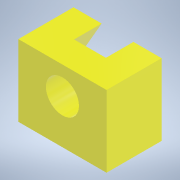
# Autodesk Inventor part: 2x 2x M6 Nut Holder
Saved by Autodesk Inventor 2022 (Build 260153000, 153)
## iProperties
Created: 2021-06-21
Part Number: 2x 2x M6 Nut Holder
Material: ABS Plastic
Document SubType Name: Modeling
Designer: benka
Density: 1.06 g/cm^3
Appearance: Yellow
Author: benka
Autodesk Inventor part; units mm, degrees
ref_plane "YZ Plane" through (0, 0, 0) normal (1, 0, 0) x (0, 1, 0)
ref_plane "XZ Plane" through (0, 0, 0) normal (0, 1, 0) x (-1, 0, 0)
ref_plane "XY Plane" through (0, 0, 0) normal (0, 0, 1) x (1, 0, 0)
sketch "Sketch1" plane through (0, 1.5, 0) normal (0, 0, 1) x (1, 0, 0)
  line L0 (8, 5) -> (8, -8)
  line L1 (8, -8) -> (-8, -8)
  line L2 (-8, -8) -> (-8, 5)
  line L3 (-8, 5) -> (8, 5)
  line L4 (-4.3301, 2.5) -> (-5.7735, 0)
  line L5 (-5.7735, 0) -> (-4.3301, -2.5)
  line L6 (-4.3301, -2.5) -> (-2.8868, -5)
  line L7 (-2.8868, -5) -> (0, -5)
  line L8 (0, -5) -> (2.8868, -5)
  line L9 (2.8868, -5) -> (4.3301, -2.5)
  line L10 (4.3301, -2.5) -> (5.7735, 0)
  line L11 (5.7735, 0) -> (4.3301, 2.5)
  line L12 (4.3301, 2.5) -> (2.8868, 5)
  line L13 (-2.8868, 5) -> (-4.3301, 2.5)
  point P0 (0, 0)
  constraints: 28 end point, 1 parallel, 1 perpendicular
extrude "Extrusion1" add sketch "Sketch1" along normal blind 5 contours L0 L1 L2 L3 L13 L4 L5 L6 L7 L8 L9 L10 L11 L12
sketch "Sketch2" plane through (0, 1.5, 5) normal (0, 0, 1) x (1, 0, 0)
  line L0 (-8, 5) -> (-8, -8) projected
  line L1 (8, 5) -> (-8, 5) projected
  line L2 (8, -8) -> (8, 5) projected
  line L3 (-8, -8) -> (8, -8) projected
  circle A0 centre (0, 0) radius 3 projected
extrude "Extrusion2" add sketch "Sketch2" along normal blind 5
body "Solid1"
